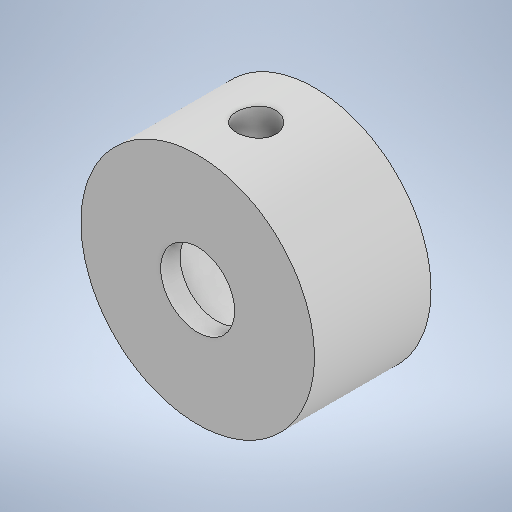
# Autodesk Inventor part: SuspensionLock
Saved by Autodesk Inventor 2025.2 (Build 292293000, 293)
## iProperties
Created: 2025-01-06
Part Number: SuspensionLock
Material: 일반
Document SubType Name: Modeling
Designer: SEON
Density: 1 g/cm^3
Appearance: 기본값
Author: SEON
Autodesk Inventor part; units mm, degrees
ref_plane "YZ Plane" through (0, 0, 0) normal (1, 0, 0) x (0, 1, 0)
ref_plane "XY Plane" through (0, 0, 0) normal (0, 0, 1) x (1, 0, 0)
sketch "스케치1" plane through (0, 0, 0) normal (0, 0, 1) x (1, 0, 0)
  circle A0 centre (0, 0) radius 4
  circle A1 centre (0, 0) radius 6
  circle A2 centre (0, 0) radius 1.9
  dimension "d0" = 8
  dimension "d1" = 2
  dimension "d11" = 3.8
  constraints: 3 centre point, 2 coincident
  measures "d0" diameter of A0
  measures "d1" radial gap between concentric circles of A0 A1
  measures "d11" diameter of A2
extrude "돌출1" add sketch "스케치1" along normal blind 1 contours A0 | A1
extrude "돌출2" add sketch "스케치1" against normal blind 5 contours A1
ref_plane "작업 평면1" through (0, 6, 0) normal (0, 1, 0) x (-1, 0, 0)
sketch "스케치2" plane through (0, 6, 0) normal (0, 1, 0) x (-1, 0, 0)
  circle A0 centre (0, -2) radius 1
  line L0 (-6, -5) -> (6, -5) projected
  line L1 (-4, 0) -> (4, 0) projected
  point P0 (0, 0)
  dimension "d6" = 2
  dimension "d10" = 2
  constraints: 1 centre point, 1 vertical alignment
  measures "d6" diameter of A0
  measures "d10" distance from line of A0.centre L1
extrude "돌출3" cut sketch "스케치2" against normal through all
